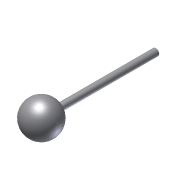
# Autodesk Inventor part: JointD2
Saved by Autodesk Inventor 2011 SP1 (Build 150282100, 282)
## iProperties
Created: 2012-10-24
Part Number: JointD2
Document SubType Name: Modeling
Designer: arihon
Density: 1 g/cm^3
Author: arihon
Autodesk Inventor part; units mm, degrees
ref_plane "YZ Plane" through (0, 0, 0) normal (1, 0, 0) x (0, 1, 0)
ref_plane "XZ Plane" through (0, 0, 0) normal (0, 1, 0) x (-1, 0, 0)
ref_plane "XY Plane" through (0, 0, 0) normal (0, 0, 1) x (1, 0, 0)
sketch "スケッチ1" plane through (0, 0, 0) normal (0, 0, 1) x (1, 0, 0)
  arc A0 (0, 7.5) -> (0, -7.5) centre (0, 0) ccw
  line L0 (0, 0) -> (-1.5, 0)
  line L1 (-1.5, 0) -> (-1.5, 50)
  line L2 (-1.5, 50) -> (0, 50)
  line L3 (0, 50) -> (0, 0)
  line L4 (0, -7.5) -> (0, 0)
  arc A1 (0, -7.5) -> (0, 7.5) centre (0, 0) ccw
  dimension "d0" = 15
  dimension "d1" = 1.5
  dimension "d2" = 50
  constraints: 10 end point, 4 point on circle, 2 centre point, 2 parallel, 1 coincident, 1 collinear, 1 horizontal, 1 perpendicular, 1 point on line
  measures "d0" diameter of A0
  measures "d1" distance of L1.end L2.end
  measures "d2" distance of L0.end L1.end
revolve "回転1" add sketch "スケッチ1" angle 360 about axis through (0, 50, 0) along (0, -1, 0) contours L3 L0 L1 A0 | A0 L1 L2 L3 | L1 L0 L4 A0
